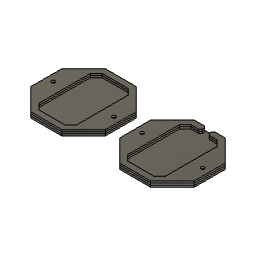
Lamp_Base v3 (Autodesk Fusion 360 design; units mm, degrees)
Autodesk Fusion 360 part; units mm, degrees
note: some values were not read from the file. Chosen so that the rebuilt part matches the saved one: which face or edge a step refers to.
sketch "Sketch1" plane through (0, 0, 0) normal (0, 0, 1) x (1, 0, 0)
  line L0 (0, 0) -> (130, 0)
  line L1 (130, 0) -> (130, 130)
  line L2 (130, 130) -> (0, 130)
  line L3 (0, 130) -> (0, 0)
  dimension "d1" = 130
  constraint horizontal L0
  constraint vertical L1
  constraint horizontal L2
  constraint vertical L3
  constraint coincident L0.start L3.end
  constraint equal L1 L2
  measures "d1" distance of L0.start L2.end
extrude "Extrude1" add sketch "Sketch1" along normal blind 3.175 makes body 1
chamfer "Chamfer1" distance 38.07 angle 45 4 edges at (130, 0, 1.5875) (0, 0, 1.5875) (130, 130, 1.5875) (0, 130, 1.5875) measured on face at (86.6667, 0, 2.1167) measured on face at (0, 43.3333, 2.1167) measured on face at (130, 86.6667, 2.1167) measured on face at (43.3333, 130, 2.1167) on bodies 1
sketch "Sketch2" plane through (0, 0, 3.175) normal (0, 0, 1) x (-1, 0, 0)
  line L0 (-38.07, -130) -> (0, -91.93)
  line L1 (0, -91.93) -> (0, -38.07)
  line L2 (0, -38.07) -> (-38.07, 0)
  line L3 (-38.07, 0) -> (-91.93, 0)
  line L4 (-91.93, 0) -> (-130, -38.07)
  line L5 (-130, -38.07) -> (-130, -91.93)
  line L6 (-130, -91.93) -> (-91.93, -130)
  line L7 (-91.93, -130) -> (-38.07, -130)
copy_body "CopyPasteBodies1" bodies 1 makes body 2
move_body "Move1" bodies 2 to x (1, 0, 0) y (0, 1, 0) z (0, 0, 1) at (170, 0, 0)
shell "Shell1" thickness 10 removed faces 2 at (73.9767, 86.6667, 3.175) at (73.9767, 86.6667, 0) on bodies 1
sketch "Sketch3" plane through (0, 0, 0) normal (0, 0, -1) x (1, 0, 0)
  line L0 (10, -42.2121) -> (42.2121, -10)
  line L1 (42.2121, -10) -> (87.7879, -10)
  line L2 (87.7879, -10) -> (120, -42.2121)
  line L3 (120, -42.2121) -> (120, -87.7879)
  line L4 (120, -87.7879) -> (87.7879, -120)
  line L5 (87.7879, -120) -> (42.2121, -120)
  line L6 (42.2121, -120) -> (10, -87.7879)
  line L7 (10, -87.7879) -> (10, -42.2121)
  line L8 (0, -91.93) -> (38.07, -130)
  line L9 (38.07, -130) -> (91.93, -130)
  line L10 (91.93, -130) -> (130, -91.93)
  line L11 (130, -91.93) -> (130, -38.07)
  line L12 (130, -38.07) -> (91.93, 0)
  line L13 (91.93, 0) -> (38.07, 0)
  line L14 (38.07, 0) -> (0, -38.07)
  line L15 (0, -38.07) -> (0, -91.93)
  line L16 (59, -120) -> (71, -120)
  line L17 (71, -120) -> (71, -130)
  line L18 (71, -130) -> (59, -130)
  line L19 (59, -130) -> (59, -120)
  line L20 (65, -120) -> (65, -130) construction
  line L21 (65, -120) -> (65, -130) construction
  dimension "d7" = 12
  constraint horizontal L16
  constraint vertical L17
  constraint horizontal L18
  constraint vertical L19
  constraint coincident L9 L17.end
  constraint coincident L5 L16.start
  constraint midpoint L5 L20.start
  constraint midpoint L9 L20.end
  constraint midpoint L16 L20.start
  constraint midpoint L18 L20.end
  constraint coincident L20.start L21.start
  measures "d7" distance of L16.start L16.end
extrude "Extrude2" cut sketch "Sketch3" against normal blind 5 contours L5 L9 L16 L17 L18 L19 bodies 1
chamfer "Chamfer2" distance 3 angle 45 4 edges at (59, 130, 1.5875) (71, 130, 1.5875) (71, 120, 1.5875) (59, 120, 1.5875) on bodies 1
sketch "Sketch5" plane through (0, 0, 0) normal (0, 0, -1) x (1, 0, 0)
  line L0 (59, -123) -> (56, -120)
  line L1 (56, -120) -> (42.2121, -120)
  line L2 (42.2121, -120) -> (10, -87.7879)
  line L3 (10, -87.7879) -> (10, -42.2121)
  line L4 (10, -42.2121) -> (42.2121, -10)
  line L5 (42.2121, -10) -> (87.7879, -10)
  line L6 (87.7879, -10) -> (120, -42.2121)
  line L7 (120, -42.2121) -> (120, -87.7879)
  line L8 (120, -87.7879) -> (87.7879, -120)
  line L9 (87.7879, -120) -> (74, -120)
  line L10 (74, -120) -> (71, -123)
  line L11 (71, -123) -> (71, -127)
  line L12 (71, -127) -> (74, -130)
  line L13 (74, -130) -> (91.93, -130)
  line L14 (91.93, -130) -> (130, -91.93)
  line L15 (130, -91.93) -> (130, -38.07)
  line L16 (130, -38.07) -> (91.93, 0)
  line L17 (91.93, 0) -> (38.07, 0)
  line L18 (38.07, 0) -> (0, -38.07)
  line L19 (0, -38.07) -> (0, -91.93)
  line L20 (0, -91.93) -> (38.07, -130)
  line L21 (38.07, -130) -> (56, -130)
  line L22 (56, -130) -> (59, -127)
  line L23 (59, -127) -> (59, -123)
sketch "Sketch6" plane through (0, 0, 0) normal (0, 0, -1) x (1, 0, 0)
  line L0 (170, -91.93) -> (208.07, -130)
  line L1 (208.07, -130) -> (261.93, -130)
  line L2 (261.93, -130) -> (300, -91.93)
  line L3 (300, -91.93) -> (300, -38.07)
  line L4 (300, -38.07) -> (261.93, 0)
  line L5 (261.93, 0) -> (208.07, 0)
  line L6 (208.07, 0) -> (170, -38.07)
  line L7 (170, -38.07) -> (170, -91.93)
copy_body "Body->Comp1" bodies 2 removing the originals makes body 3 in component "Base"
copy_body "Body->Comp2" bodies 1 removing the originals makes body 4 in component "frame"
sketch "Sketch7" plane through (0, 0, 6.35) normal (0, 0, 1) x (-1, 0, 0)
  line L0 (-226, -120) -> (-229, -123)
  line L1 (-229, -123) -> (-229, -127)
  line L2 (-229, -127) -> (-226, -130)
  line L3 (-226, -130) -> (-208.07, -130)
  line L4 (-208.07, -130) -> (-170, -91.93)
  line L5 (-170, -91.93) -> (-170, -38.07)
  line L6 (-170, -38.07) -> (-208.07, 0)
  line L7 (-208.07, 0) -> (-261.93, 0)
  line L8 (-261.93, 0) -> (-300, -38.07)
  line L9 (-300, -38.07) -> (-300, -91.93)
  line L10 (-300, -91.93) -> (-261.93, -130)
  line L11 (-261.93, -130) -> (-244, -130)
  line L12 (-244, -130) -> (-241, -127)
  line L13 (-241, -127) -> (-241, -123)
  line L14 (-241, -123) -> (-244, -120)
  line L15 (-244, -120) -> (-257.7879, -120)
  line L16 (-257.7879, -120) -> (-290, -87.7879)
  line L17 (-290, -87.7879) -> (-290, -42.2121)
  line L18 (-290, -42.2121) -> (-257.7879, -10)
  line L19 (-257.7879, -10) -> (-212.2121, -10)
  line L20 (-212.2121, -10) -> (-180, -42.2121)
  line L21 (-180, -42.2121) -> (-180, -87.7879)
  line L22 (-180, -87.7879) -> (-212.2121, -120)
  line L23 (-212.2121, -120) -> (-226, -120)
  line L24 (-257.7879, -10) -> (-257.7879, -120)
  line L25 (-212.2121, -120) -> (-212.2121, -10)
  constraint coincident L18.end L19.start
  constraint coincident L15.end L16.start
  constraint coincident L22.end L23.start
  constraint coincident L19.end L20.start
sketch "Sketch8" plane through (0, 0, 6.35) normal (0, 0, 1) x (-1, 0, 0)
  line L0 (-226, -120) -> (-229, -123)
  line L1 (-229, -123) -> (-229, -127)
  line L2 (-229, -127) -> (-226, -130)
  line L3 (-226, -130) -> (-208.07, -130)
  line L4 (-208.07, -130) -> (-170, -91.93)
  line L5 (-170, -91.93) -> (-170, -38.07)
  line L6 (-170, -38.07) -> (-208.07, 0)
  line L7 (-208.07, 0) -> (-261.93, 0)
  line L8 (-261.93, 0) -> (-300, -38.07)
  line L9 (-300, -38.07) -> (-300, -91.93)
  line L10 (-300, -91.93) -> (-261.93, -130)
  line L11 (-261.93, -130) -> (-244, -130)
  line L12 (-244, -130) -> (-241, -127)
  line L13 (-241, -127) -> (-241, -123)
  line L14 (-241, -123) -> (-244, -120)
  line L15 (-244, -120) -> (-257.7879, -120)
  line L16 (-257.7879, -120) -> (-290, -87.7879)
  line L17 (-290, -87.7879) -> (-290, -42.2121)
  line L18 (-290, -42.2121) -> (-257.7879, -10)
  line L19 (-257.7879, -10) -> (-212.2121, -10)
  line L20 (-212.2121, -10) -> (-180, -42.2121)
  line L21 (-180, -42.2121) -> (-180, -87.7879)
  line L22 (-180, -87.7879) -> (-212.2121, -120)
  line L23 (-212.2121, -120) -> (-226, -120)
extrude "Extrude1'" add sketch "Sketch7" against normal blind 3.175 contours L20 L21 L22 L25 | L16 L17 L18 L24 sketch seen with x (1, 0, 0) y (0, 1, 0) z (0, 0, 1) at (-170, 0, -3.175) bodies 4 in component "frame"
move_face "OffsetFaces1" offset -10 2 faces at (42.2121, 83.3333, 1.0583) (87.7879, 46.6667, 1.0583) on bodies 4 in component "frame"
chamfer "Chamfer1'" distance 10 angle 45 4 edges at (32.2121, 120, 1.5875) (32.2121, 10, 1.5875) (97.7879, 10, 1.5875) (97.7879, 120, 1.5875) on bodies 4 in component "frame"
copy_body "CopyPasteBodies2" bodies 4 body 4 seen with x (1, 0, 0) y (0, 1, 0) z (0, 0, 1) at (170, 0, 3.175) makes body 5
move_body "Move2" bodies 5 to x (1, 0, 0) y (0, 1, 0) z (0, 0, 1) at (0, 0, 5)
copy_body "Body->Comp3" bodies 5 removing the originals makes body 6 in component "Component"
sketch "Sketch9" plane through (0, 0, 11.35) normal (0, 0, 1) x (-1, 0, 0)
  line L0 (-226, -120) -> (-229, -123)
  line L1 (-229, -123) -> (-229, -127)
  line L2 (-229, -127) -> (-226, -130)
  line L3 (-226, -130) -> (-208.07, -130)
  line L4 (-208.07, -130) -> (-170, -91.93)
  line L5 (-170, -91.93) -> (-170, -38.07)
  line L6 (-170, -38.07) -> (-208.07, 0)
  line L7 (-208.07, 0) -> (-261.93, 0)
  line L8 (-261.93, 0) -> (-300, -38.07)
  line L9 (-300, -38.07) -> (-300, -91.93)
  line L10 (-300, -91.93) -> (-261.93, -130)
  line L11 (-261.93, -130) -> (-244, -130)
  line L12 (-244, -130) -> (-241, -127)
  line L13 (-241, -127) -> (-241, -123)
  line L14 (-241, -123) -> (-244, -120)
  line L15 (-244, -120) -> (-257.7879, -120)
  line L16 (-257.7879, -120) -> (-267.7879, -110)
  line L17 (-267.7879, -110) -> (-267.7879, -20)
  line L18 (-267.7879, -20) -> (-257.7879, -10)
  line L19 (-257.7879, -10) -> (-212.2121, -10)
  line L20 (-212.2121, -10) -> (-202.2121, -20)
  line L21 (-202.2121, -20) -> (-202.2121, -110)
  line L22 (-202.2121, -110) -> (-212.2121, -120)
  line L23 (-212.2121, -120) -> (-226, -120)
  line L24 (-300, -38.07) -> (-267.7879, -110) construction
  line L25 (-300, -91.93) -> (-267.7879, -20) construction
  circle A0 centre (-287.94, -65) radius 3.15
  line L26 (-202.2121, -20) -> (-170, -91.93) construction
  line L27 (-202.2121, -110) -> (-170, -38.07) construction
  circle A1 centre (-182.06, -65) radius 3.15
  dimension "d21" = 6.3
  dimension "d22" = 6.3
  constraint coincident L8.end L9.start
  constraint coincident L16.end L17.start
  constraint coincident L9.end L10.start
  constraint coincident L17.end L18.start
  constraint coincident L25 A0.centre
  constraint coincident L24 A0.centre
  constraint coincident L20.end L21.start
  constraint coincident L4.end L5.start
  constraint coincident L21.end L22.start
  constraint coincident L5.end L6.start
  constraint coincident L27 A1.centre
  constraint coincident L26 A1.centre
  measures "d21" diameter of A0
  measures "d22" diameter of A1
extrude "Extrude1''" cut sketch "Sketch9" against normal blind 5 contours A0 | A1 bodies 6 in component "Component"
copy_body "CopyPasteBodies6" bodies 4 3 6 body 4 seen with x (1, 0, 0) y (0, 1, 0) z (0, 0, 1) at (170, 0, 3.175) body 6 seen with x (1, 0, 0) y (0, 1, 0) z (0, 0, 1) at (0, 0, -1.825) makes body 7 makes body 8 makes body 9
move_body "Move4" bodies 7 8 9 to x (1, 0, 0) y (0, 1, 0) z (0, 0, 1) at (-155, 0, 0)
sketch "Sketch10" plane through (0, 0, 9.525) normal (0, 0, 1) x (-1, 0, 0)
  circle A0 centre (-27.06, -65) radius 3.15
  circle A1 centre (-132.94, -65) radius 3.15
  line L0 (-71, -120) -> (-74, -123)
  line L1 (-74, -123) -> (-74, -127)
  line L2 (-74, -127) -> (-71, -130)
  line L3 (-71, -130) -> (-53.07, -130)
  line L4 (-53.07, -130) -> (-15, -91.93)
  line L5 (-15, -91.93) -> (-15, -38.07)
  line L6 (-15, -38.07) -> (-53.07, 0)
  line L7 (-53.07, 0) -> (-106.93, 0)
  line L8 (-106.93, 0) -> (-145, -38.07)
  line L9 (-145, -38.07) -> (-145, -91.93)
  line L10 (-145, -91.93) -> (-106.93, -130)
  line L11 (-106.93, -130) -> (-89, -130)
  line L12 (-89, -130) -> (-86, -127)
  line L13 (-86, -127) -> (-86, -123)
  line L14 (-86, -123) -> (-89, -120)
  line L15 (-89, -120) -> (-102.7879, -120)
  line L16 (-102.7879, -120) -> (-112.7879, -110)
  line L17 (-112.7879, -110) -> (-112.7879, -20)
  line L18 (-112.7879, -20) -> (-102.7879, -10)
  line L19 (-102.7879, -10) -> (-57.2121, -10)
  line L20 (-57.2121, -10) -> (-47.2121, -20)
  line L21 (-47.2121, -20) -> (-47.2121, -110)
  line L22 (-47.2121, -110) -> (-57.2121, -120)
  line L23 (-57.2121, -120) -> (-71, -120)
  line L24 (-89, -120) -> (-71, -120)
  line L25 (-71, -130) -> (-89, -130)
  constraint coincident L14.end L15.start
  constraint coincident L0.start L23.end
  constraint coincident L2.end L3.start
  constraint coincident L11.end L12.start
extrude "Extrude3" add sketch "Sketch10" against normal blind 3.175 contours L0 L1 L2 L12 L13 L14 L24 L25 bodies 9
sketch "Sketch11" plane through (0, 0, 3.175) normal (0, 0, 1) x (-1, 0, 0)
  line L0 (-53.07, -130) -> (-15, -91.93)
  line L1 (-15, -91.93) -> (-15, -38.07)
  line L2 (-15, -38.07) -> (-53.07, 0)
  line L3 (-53.07, 0) -> (-106.93, 0)
  line L4 (-106.93, 0) -> (-145, -38.07)
  line L5 (-145, -38.07) -> (-145, -91.93)
  line L6 (-145, -91.93) -> (-106.93, -130)
  line L7 (-106.93, -130) -> (-53.07, -130)
  line L8 (-89, -120) -> (-71, -120)
  line L9 (-71, -130) -> (-89, -130)
  line L10 (-74, -123) -> (-71, -120)
  line L11 (-71, -120) -> (-57.2121, -120)
  line L12 (-57.2121, -120) -> (-47.2121, -110)
  line L13 (-47.2121, -110) -> (-47.2121, -20)
  line L14 (-47.2121, -20) -> (-57.2121, -10)
  line L15 (-57.2121, -10) -> (-102.7879, -10)
  line L16 (-102.7879, -10) -> (-112.7879, -20)
  line L17 (-112.7879, -20) -> (-112.7879, -110)
  line L18 (-112.7879, -110) -> (-102.7879, -120)
  line L19 (-102.7879, -120) -> (-89, -120)
  line L20 (-89, -120) -> (-86, -123)
  line L21 (-86, -123) -> (-86, -127)
  line L22 (-86, -127) -> (-89, -130)
  line L23 (-89, -130) -> (-106.93, -130)
  line L24 (-106.93, -130) -> (-145, -91.93)
  line L25 (-145, -91.93) -> (-145, -38.07)
  line L26 (-145, -38.07) -> (-106.93, 0)
  line L27 (-106.93, 0) -> (-53.07, 0)
  line L28 (-53.07, 0) -> (-15, -38.07)
  line L29 (-15, -38.07) -> (-15, -91.93)
  line L30 (-15, -91.93) -> (-53.07, -130)
  line L31 (-53.07, -130) -> (-71, -130)
  line L32 (-71, -130) -> (-74, -127)
  line L33 (-74, -127) -> (-74, -123)
extrude "Extrude4" add sketch "Sketch11" along normal blind 3.175 contours L7 L8 L9 L10 L20 L21 L22 L32 L33 bodies 7
component "Base" placed x (1, 0, 0) y (0, 1, 0) z (0, 0, 1) at (0, 0, 0)
component "frame" placed x (1, 0, 0) y (0, 1, 0) z (0, 0, 1) at (170, 0, 3.175)
component "Component" placed x (1, 0, 0) y (0, 1, 0) z (0, 0, 1) at (0, 0, -1.825)
equation "chamfer_width = 25 mm"
